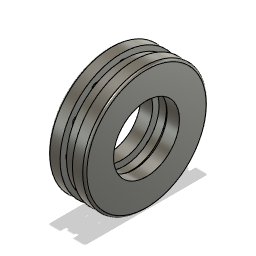
Bearing_GOST_23526-79_889000 (Autodesk Fusion 360 design; units mm, degrees)
Autodesk Fusion 360 part; units mm, degrees
sketch "Sketch1" plane through (0, 0, 0) normal (0, 0, 1) x (1, 0, 0)
  line L0 (-79.69918, 0) -> (79.69918, 0)
  line L1 (-9, 30) -> (-3, 30)
  line L2 (-3, 30) -> (-3, 15)
  line L3 (-3, 15) -> (-9, 15)
  line L4 (-9, 15) -> (-9, 30)
  line L5 (3, 30) -> (9, 30)
  line L6 (9, 30) -> (9, 16)
  line L7 (9, 16) -> (3, 16)
  line L8 (3, 16) -> (3, 30)
  line L9 (-3, 27.167) -> (3, 27.167)
  line L10 (3, 27.167) -> (3, 22.967)
  line L11 (3, 22.967) -> (-3, 22.967)
  line L12 (-3, 22.967) -> (-3, 27.167)
  line L13 (-1.8, 28.1) -> (1.8, 28.1)
  line L14 (1.8, 28.1) -> (1.8, 16.9)
  line L15 (1.8, 16.9) -> (-1.8, 16.9)
  line L16 (-1.8, 16.9) -> (-1.8, 28.1)
  line L17 (0, 28.1) -> (0, 16.9)
  line L18 (-3, 22.5) -> (3, 22.5)
  point P0 (-3, 22.5)
  point P1 (0, 27.167)
  point P2 (-1.8, 22.5)
  dimension "d1" = 18
  dimension "d2" = 32
  dimension "d3" = 30
  dimension "d4" = 60
  dimension "d5" = 60
  dimension "d6" = 3.6
  dimension "d7" = 11.2
  dimension "d9" = 6
  dimension "d18" = 0.467
  dimension "d19" = 4.667
  constraint horizontal L0
  constraint midpoint L0 origin
  constraint horizontal L1
  constraint vertical L2
  constraint horizontal L3
  constraint vertical L4
  constraint horizontal L5
  constraint vertical L6
  constraint horizontal L7
  constraint vertical L8
  constraint horizontal L9
  constraint vertical L10
  constraint horizontal L11
  constraint vertical L12
  constraint coincident L8 L10.end
  constraint coincident L2 L9.start
  constraint horizontal L13
  constraint vertical L14
  constraint horizontal L15
  constraint vertical L16
  constraint midpoint L13 L17.start
  constraint midpoint L15 L17.end
  constraint vertical origin L17.end
  constraint equal L1 L5
  constraint midpoint L9 P1
  constraint coincident L17 P1
  constraint midpoint L2 P0
  constraint coincident P0 L18.start
  constraint coincident L8 L18.end
  constraint perpendicular L8 L18
  constraint midpoint L16 P2
  constraint horizontal P0 P2
  measures "d1" distance of L4 L6
  measures "d6" distance of L13.start L13.end
  measures "d7" distance of L13.start L15.end
  measures "d9" distance of L5.start L5.end
  measures "d18" distance of L10.end L18.end
  measures "d19" distance of L9 L18.end
revolve "Revolve1" add sketch "Sketch1" angle 360 about axis through (-79.69918, 0, 0) along (1, 0, 0) contours L1 L2 L3 L4 L12 | L5 L6 L7 L8 L10 picked at (-7, 22.5) picked at (7, 22.989) makes body 1 at (-3, 24.888308, -1.490423) makes body 2 at (9, 25.162073, -2.285315)
revolve "Revolve2" add sketch "Sketch1" angle 360 about axis through (0, 28.1, 0) along (0, -1, 0) separate body contours L2 L9 L11 L12 L16 | L9 L11 L16 L17 picked at (-2.2, 24.367) picked at (-0.6, 24.367) makes body 3
revolve "Revolve3" add sketch "Sketch1" angle 360 about axis through (-79.69918, 0, 0) along (1, 0, 0) separate body contours L9 L13 L16 L17 | L9 L11 L16 L17 | L11 L16 L17 L18 | L9 L13 L14 L17 | L9 L11 L14 L17 | L15 L16 L17 L18 | L11 L14 L17 L18 | L14 L15 L17 L18 picked at (-1.2, 27.789) picked at (-0.6, 24.367) picked at (-1.2, 22.811333) picked at (0.6, 27.789) picked at (1.2, 24.367) picked at (-1.2, 18.766667) picked at (0.6, 22.811333) picked at (0.6, 18.766667) makes body 4
pattern_circular "C-Pattern1" count 12 over 360 about axis through (1.75, 0, 0) along (1, 0, 0) of bodies 3 makes body 5 at (-2.985092, 20.953089, 12.442185) makes body 6 at (-2.985092, 11.924815, 21.251793) makes body 7 at (-2.985092, -0.298704, 24.367) makes body 8 at (-2.985092, -12.442185, 20.953089) makes body 9 at (-2.996271, -22.389645, 12.753997) makes body 10 at (-2.985092, -24.367, -0.298704) makes body 11 at (-2.985092, -20.953089, -12.442185) makes body 12 at (-2.996271, -12.753997, -22.389645) makes body 13 at (-2.985092, 0.298704, -24.367) makes body 14 at (-2.996271, 13.013003, -22.240108) makes body 15 at (-2.985092, 21.251793, -11.924815)
fillet "Fillet1" radius 1 2 edges at (-9, -10.848463, 27.96982) (9, -10.848463, 27.96982) on bodies 1 2
ref_plane "WorkPlane1" through (0, 0, 0) normal (0, -0.207912, 0.978148) x (1, 0, 0)
sketch "Sketch2" plane through (0, 0, 0) normal (0, -0.207912, 0.978148) x (1, 0, 0)
  line L0 (-3, 18.333) -> (3, 18.333)
  line L1 (3, 18.333) -> (3, 22.533)
  line L2 (3, 22.533) -> (-3, 22.533)
  line L3 (-3, 22.533) -> (-3, 18.333)
  line L4 (0, 18.333) -> (0, 22.533)
  point P0 (0, 18.333)
  dimension "d20" = 18.333
  dimension "d21" = 4.2
  dimension "d22" = 6
  constraint horizontal L0
  constraint vertical L1
  constraint horizontal L2
  constraint vertical L3
  constraint midpoint L0 P0
  constraint coincident P0 L4.start
  constraint midpoint L2 L4.end
  constraint vertical origin L4.start
  measures "d20" vertical distance of L0.end origin
  measures "d21" distance of L0.end L1.end
  measures "d22" distance of L1.end L2.end
revolve "Revolve4" add sketch "Sketch2" angle 360 about axis through (0, 17.93238, 3.811645) along (0, 0.978148, 0.207912) separate body contours L0 L2 L3 L4 picked at (-1, 19.733) makes body 16
pattern_circular "C-Pattern2" count 12 over 360 about axis through (1.75, 0, 0) along (1, 0, 0) of bodies 16 makes body 17 at (-2.996271, 15.80494, 14.029609) makes body 18 at (-2.996271, 6.240051, 18.720989) makes body 19 at (-2.985092, -3.810545, 19.363891) makes body 20 at (-2.996271, -14.029609, 15.80494) makes body 21 at (-2.985092, -20.006373, 6.81454) makes body 22 at (-2.985092, -19.363891, -3.810545) makes body 23 at (-2.996271, -14.764537, -13.092826) makes body 24 at (-2.985092, -6.381916, -18.674894) makes body 25 at (-2.985092, 3.810545, -19.363891) makes body 26 at (-2.996271, 13.092826, -14.764537) makes body 27 at (-2.996271, 20.052468, -6.672675)
